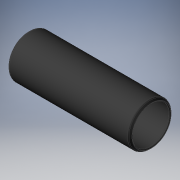
# Autodesk Inventor part: 04R-2.25550C
Saved by Autodesk Inventor 2019 (Build 230136000, 136)
## iProperties
Created: 2023-02-26
Part Number: 04R-2.25550C
Material: Generic
Catalog Web Link: www.cadenas.de
Description: Tube-Original Line - Standard Air Cylinders
Vendor: BIMBA
Document SubType Name: Modeling
Designer: psAdmin
Manufacturer: BIMBA
Mass: 2.17676 g
Surface Area: 74.325 cm^2
Volume: 2.17676 cm^3
Density: 1 g/cm^3
Appearance: PSOLRGB-180-180-180
Category: PARTsolutions
Company: BIMBA
Title: 04R-2.25550C
Author: Cadenas PARTsolutions
Comments: Original Line - Standard Air Cylinders
PSOL_IDENT_0: {$CADENAS_DATA/23d-libs/bimba/bimba_brand/bimba_imperial/bimba_full_line/original_line_cylinders/sta
PSOL_IDENT_1: ndard_air_cylinders/tube.prj},203 {VTYP=3D},{NB=04R-2.25550C},{LINA=04R-2.25550C},{NN=Tube},{DATE=26
PSOL_IDENT_2: .01.2023 11:43:57},{GEOMDATE=25.01.2023 10:00:00},{VERSION=},{LINEID=40},{WBVAR=MNT,ACTING,NR,L,FOUR
PSOL_IDENT_3: HOLES,SR,K},{WBNUMERIC=L,FOURHOLES}  {NB=04R-2.25550C},{LINA=04R-2.25550C},{KT=DUMMY},{PN=04R-2.2555
PSOL_IDENT_4: 0C},{BORE=0.75000000},{BOREPN=04},{MNT=},{MNTALG='' , 'Front Nose' , 'BF' , 'Front Block' , 'BFT' , '
PSOL_IDENT_5: Front Trunnion' , 'A' , 'Adjustable Stroke'},{ACTING=R},{ACTINGALG= '' , 'Single Acting' , 'R' , 'Re
PSOL_IDENT_6: verse/Double Acting' },{NR=},{NRALG= '' , 'N/A' },{L=2.2555},{OD=0.8075},{ODN=0.8050},{ODP=0.8625},{
PSOL_IDENT_7: ODB=0.8325},{ID=0.7615},{DV=0.00000000},{LV=0.00000000},{LV1=0.00000000},{G=0.0300},{FOURHOLES=0},{A
PSOL_IDENT_8: A=0.3750},{BB=0.0940},{SR=C},{SRALG= 'C' , 'Carbon Steel Rod' , 'SR' , '303 Stainless Steel Rod' , ''
PSOL_IDENT_9: , '303 Stainless Steel Rod'},{KALG= '', 'Standard' , 'K' , 'Ports Rotated 90deg' },{K=}
NB: 04R-2.25550C
NN: Tube
NT: Original Line - Standard Air Cylinders
NBSYN: $PN.
LINA: 04R-2.25550C
CATALOG: Bimba Products
BORE: 0
BOREPN: 04
MNT: Front Nose
MNTALG: '' , 'Front Nose' , 'BF' , 'Front Block' , 'BFT' , 'Front Trunnion' , 'A' , 'Adjustable Stroke'
ACTING: Reverse/Double Acting
NR: N/A
L: 2.2555
ODN: 0.805
ODP: 0.8625
ODB: 0.8325
ID: 0.7615
DV: 0
LV: 0
LV1: 0
G: 0.03
FOURHOLES: 0
AA: 0.375
BB: 0.094
SR: Carbon Steel Rod
K: Standard
SUPPLIER: BIMBA
ARTICLENO: 04R-2.25550C
BOMINFO: 04R-2.25550C
CREATOR: CADENAS GmbH
Autodesk Inventor part; units mm, degrees
sketch "Sketch_1" plane through (0, 0, 0) normal (0, 0, 1) x (1, 0, 0)
  line L0 (57.2897, 0) -> (0, 0)
  arc A0 (-0.6395, 9.3472) -> (-0.6395, 9.1676) centre (-0.5497, 9.2574) ccw
  line L1 (-0.6395, 9.1676) -> (-0.381, 8.9091)
  line L2 (-0.381, 8.9091) -> (0, 8.9091)
  line L3 (0, 8.9091) -> (0.762, 9.671)
  line L4 (0.762, 9.671) -> (56.5277, 9.671)
  line L5 (56.5277, 9.671) -> (57.2897, 8.9091)
  line L6 (57.2897, 8.9091) -> (57.6707, 8.9091)
  line L7 (57.6707, 8.9091) -> (57.9292, 9.1676)
  arc A1 (57.9292, 9.1676) -> (57.9292, 9.3472) centre (57.8394, 9.2574) ccw
  line L8 (57.9292, 9.3472) -> (57.2443, 10.0321)
  arc A2 (57.2443, 10.0321) -> (56.7055, 10.2553) centre (56.7055, 9.4933) ccw
  line L9 (56.7055, 10.2553) -> (0.5842, 10.2553)
  arc A3 (0.5842, 10.2553) -> (0.0454, 10.0321) centre (0.5842, 9.4933) ccw
  line L10 (0.0454, 10.0321) -> (-0.6395, 9.3472)
  constraints: 22 end point, 8 point on circle, 4 centre point
revolve "Revolution1" add sketch "Sketch_1" angle 360 about axis through (57.2897, 0, 0) along (1, 0, 0)
ref_plane "cp1_XY" through (28.6449, 0, 10.2553) normal (1, 0, 0) x (0, 0, -1)
ref_plane "cp1_YZ" through (28.6449, 0, 10.2553) normal (0, 0, -1) x (0, 1, 0)
ref_plane "cp1_ZX" through (28.6449, 0, 10.2553) normal (0, 1, 0) x (1, 0, 0)
ref_plane "cp2_XY" through (28.6449, -10.2553, 0) normal (1, 0, 0) x (0, 0, -1)
ref_plane "cp2_YZ" through (28.6449, -10.2553, 0) normal (0, 0, -1) x (0, 1, 0)
ref_plane "cp2_ZX" through (28.6449, -10.2553, 0) normal (0, 1, 0) x (1, 0, 0)
ref_plane "cp3_XY" through (28.6449, 0, -10.2553) normal (1, 0, 0) x (0, 0, -1)
ref_plane "cp3_YZ" through (28.6449, 0, -10.2553) normal (0, 0, -1) x (0, 1, 0)
ref_plane "cp3_ZX" through (28.6449, 0, -10.2553) normal (0, 1, 0) x (1, 0, 0)
ref_plane "cp4_XY" through (28.6449, 10.2553, 0) normal (1, 0, 0) x (0, 0, -1)
ref_plane "cp4_YZ" through (28.6449, 10.2553, 0) normal (0, 0, -1) x (0, 1, 0)
ref_plane "cp4_ZX" through (28.6449, 10.2553, 0) normal (0, 1, 0) x (1, 0, 0)
ref_plane "tube_front_XY" through (0, 0, 0) normal (1, 0, 0) x (0, 0, -1)
ref_plane "tube_front_YZ" through (0, 0, 0) normal (0, 0, -1) x (0, 1, 0)
ref_plane "tube_front_ZX" through (0, 0, 0) normal (0, 1, 0) x (1, 0, 0)
ref_plane "tube_rear_XY" through (57.2897, 0, 0) normal (1, 0, 0) x (0, 0, -1)
ref_plane "tube_rear_YZ" through (57.2897, 0, 0) normal (0, 0, -1) x (0, 1, 0)
ref_plane "tube_rear_ZX" through (57.2897, 0, 0) normal (0, 1, 0) x (1, 0, 0)
body "Solid1"
